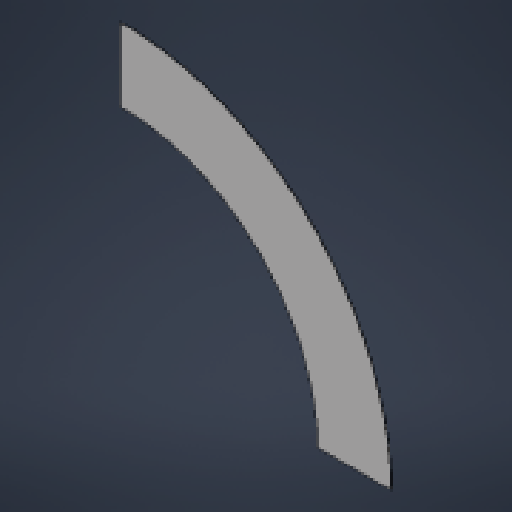
# Autodesk Inventor part: 3DPRINT,CABLE,TRAY
Saved by Autodesk Inventor 2026.1 (Build 301233020, 233B)
## iProperties
Created: 2026-02-14
Part Number: 3DPRINT,CABLE,TRAY
Material: Generic
Document SubType Name: Modeling
Designer: Owen L
Density: 1 g/cm^3
Appearance: Default
Author: Owen L
Autodesk Inventor part; units mm, degrees
ref_plane "YZ Plane" through (0, 0, 0) normal (1, 0, 0) x (0, 1, 0)
ref_plane "XZ Plane" through (0, 0, 0) normal (0, 1, 0) x (-1, 0, 0)
ref_plane "XY Plane" through (0, 0, 0) normal (0, 0, 1) x (1, 0, 0)
sketch "Sketch1" plane through (0, 0, 0) normal (0, 0, 1) x (1, 0, 0)
  arc A0 (187.325, 0) -> (0, 187.325) centre (0, 0) ccw
  arc A1 (136.525, 0) -> (0, 136.525) centre (0, 0) ccw
  line L0 (0, 136.525) -> (0, 187.325)
  line L1 (136.525, 0) -> (187.325, 0)
  point P0 (161.925, 0)
  point P1 (0, 161.925)
  dimension "d2" = 187.325
  dimension "d3" = 136.525
  constraints: 4 end point, 4 point on circle, 2 centre point, 2 coincident, 2 midpoint, 1 horizontal alignment, 1 perpendicular, 1 vertical, 1 vertical alignment
  measures "d2" radius of A0
  measures "d3" radius of A1
extrude "Extrusion1" add sketch "Sketch1" along normal blind 0.4
body "Solid1"
